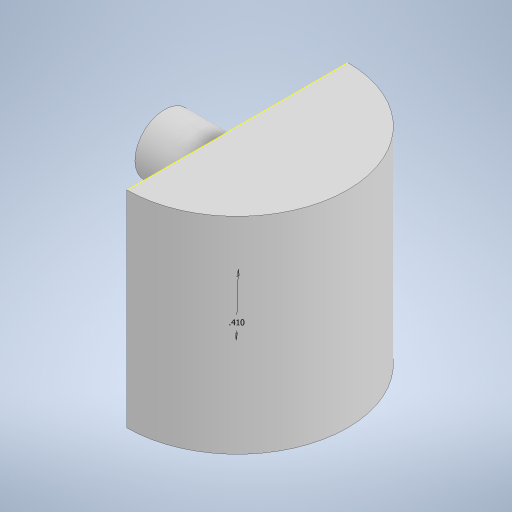
# Autodesk Inventor part: Piston Mold
Saved by Autodesk Inventor 2023 (Build 270158000, 158)
## iProperties
Created: 2022-11-15
Part Number: Piston Mold
Material: Generic
Document SubType Name: Modeling
Designer: tommy
Density: 1 g/cm^3
Appearance: Default
Author: tommy
Autodesk Inventor part; units mm, degrees
ref_plane "YZ Plane" through (0, 0, 0) normal (1, 0, 0) x (0, 1, 0)
ref_plane "XZ Plane" through (0, 0, 0) normal (0, 1, 0) x (-1, 0, 0)
ref_plane "XY Plane" through (0, 0, 0) normal (0, 0, 1) x (1, 0, 0)
sketch "Sketch1" plane through (0, 0, 0) normal (0, 1, 0) x (-1, 0, 0)
  arc A0 (0, 19.05) -> (0, -19.05) centre (0, 0) ccw
  line L0 (0, 19.05) -> (0, -19.05)
  dimension "d0" = 38.1
  constraints: 2 end point, 2 point on circle, 1 centre point, 1 coincident, 1 vertical
  measures "d0" diameter of A0
extrude "Extrusion1" add sketch "Sketch1" along normal blind 35.56
sketch "Sketch2" plane through (0, 0, -19.05) normal (-1, 0, 0) x (0, 0, 1)
  line L0 (0, 35.56) -> (38.1, 35.56) projected
  line L1 (0, 0) -> (0, 35.56) projected
  circle A0 centre (19.05, 26.67) radius 5.08
  circle A1 centre (19.05, 8.89) radius 5.207
  point P0 (19.05, 0)
  dimension "d6" = 10.414
  constraints: 2 centre point
  measures "d6" diameter of A1
extrude "Extrusion2" cut sketch "Sketch2" against normal blind 12.7 contours A1
extrude "Extrusion3" add sketch "Sketch2" along normal blind 12.573 contours A0
body "Solid1"
